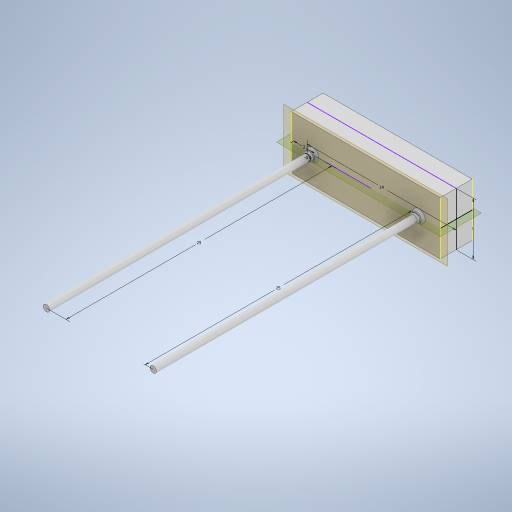
# Autodesk Inventor part: A54
Saved by Autodesk Inventor 2024 (Build 280153000, 153)
## iProperties
Created: 2023-12-15
Part Number: A54
Material: Generic
Document SubType Name: Sheet Metal
Designer: user
Density: 1 g/cm^3
Sheet Metal Rule: Default
Appearance: Default
Author: user
Autodesk Inventor part; units mm, degrees
ref_plane "YZ Plane" through (0, 0, 0) normal (1, 0, 0) x (0, 1, 0)
ref_plane "XZ Plane" through (0, 0, 0) normal (0, 1, 0) x (-1, 0, 0)
ref_plane "XY Plane" through (0, 0, 0) normal (0, 0, 1) x (1, 0, 0)
sketch "Sketch1" plane through (0, 0, 0) normal (0, 0, 1) x (1, 0, 0)
  line L0 (0, 0) -> (14, 0)
  line L1 (14, 0) -> (14, 5)
  line L2 (14, 5) -> (0, 5)
  line L3 (0, 5) -> (0, 0)
  dimension "d39" = 14
  dimension "d40" = 5
  constraints: 8 end point, 1 horizontal, 1 perpendicular
  measures "d39" distance of L0.start L0.end
  measures "d40" distance of L0.end L1.end
extrude "Extrusion1" add sketch "Sketch1" along normal mid plane 3
ref_plane "Work Plane5" through (0, 0, 1.5) normal (0, 0, 1) x (1, 0, 0)
sketch "Sketch9" plane through (0, 0, 1.5) normal (0, 0, 1) x (1, 0, 0)
  line L0 (0, 5) -> (0, 0) projected
  line L1 (0, 2.5) -> (2, 2.5)
  line L2 (14, 0) -> (14, 5) projected
  line L3 (14, 2.5) -> (12, 2.5)
  circle A0 centre (12, 2.5) radius 0.4
  circle A1 centre (2, 2.5) radius 0.4
  dimension "d43" = 2
  dimension "d44" = 2
  dimension "d45" = 0.8
  dimension "d46" = 0.8
  constraints: 4 end point, 2 centre point, 2 coincident, 2 horizontal, 2 midpoint
  measures "d43" distance of L1.start L1.end
  measures "d44" distance of L3.start L3.end
  measures "d45" diameter of A0
  measures "d46" diameter of A1
extrude "Extrusion5" add sketch "Sketch9" along normal blind 0.5
fillet "Fillet5" radius 0.2 4 edges at (11.6, 2.5, 1.5) (11.6, 2.5, 2) (1.6, 2.5, 1.5) (1.6, 2.5, 2)
sketch "Sketch10" plane through (14, 0, 1.5) normal (1, 0, 0) x (0, 0, -1)
  line L0 (3, 5) -> (3, 0) projected
  line L1 (3, 2.5) -> (0, 2.5)
  line L2 (0, 0) -> (0, 5) projected
  point P0 (1.5, 0)
  constraints: 2 end point, 2 midpoint
sketch "Sketch11" plane through (0, 0, 1.5) normal (0, 0, 1) x (1, 0, 0)
  line L0 (14, 0) -> (14, 5) projected
  circle A0 centre (12, 2.5) radius 0.2 projected
  line L1 (7.4995, 2.5) -> (3.1588, 2.5)
  point P0 (0, 0)
  constraints: 2 end point
sketch "Sketch12" plane through (0, 0, 1.5) normal (-1, 0, 0) x (0, 0, 1)
  line L0 (-3, 5) -> (-3, 0) projected
  line L1 (-3, 2.5) -> (0, 2.5)
  line L2 (0, 1.9) -> (0, 3.1) projected
  point P0 (-1.5, 0)
  constraints: 2 end point, 2 midpoint
sketch "Sketch13" plane through (0, 0, 1.5) normal (0, 0, 1) x (1, 0, 0)
  line L0 (0, 5) -> (0, 0) projected
  point P0 (0, 2.5)
  constraints: 1 midpoint
ref_plane "Work Plane7" through (2, 2.5, 2) normal (0, 0, 1) x (1, 0, 0)
ref_plane "Work Plane8" through (12, 2.5, 2) normal (0, 0, 1) x (1, 0, 0)
sketch "Sketch15" plane through (2, 2.5, 2) normal (0, 0, 1) x (1, 0, 0)
  circle A0 centre (0, 0) radius 0.2 projected
  circle A1 centre (0, 0) radius 0.3
  point P0 (-2, -2.5)
  dimension "d57" = 0.6
  constraints: 1 centre point, 1 coincident
  measures "d57" diameter of A1
sketch "Sketch17" plane through (12, 2.5, 2) normal (0, 0, 1) x (1, 0, 0)
  circle A0 centre (0, 0) radius 0.3
  point P0 (-12, -2.5)
  dimension "d63" = 0.6
  constraints: 1 centre point
  measures "d63" diameter of A0
ref_plane "Work Plane9" through (0, 2.5, -1.5) normal (0, -1, 0) x (0, 0, 1)
sketch "Sketch18" plane through (0, 2.5, -1.5) normal (0, -1, 0) x (0, 0, 1)
  line L0 (3, -2) -> (28, -2)
  line L1 (2.9646, -12) -> (27.9646, -12)
  point P0 (1.5, 0)
  point P1 (3, 0)
  dimension "d66" = 2
  dimension "d67" = 25
  dimension "d69" = 25
  constraints: 4 end point
  measures "d66" distance of point (3, 0) L0.start
  measures "d67" distance of L0.start L0.end
  measures "d69" distance of L1.start L1.end
sweep "Sweep6" add profiles "Sketch15" path "Sketch18" path curves L0 contours A0 | A1
sweep "Sweep7" add profiles "Sketch17" path "Sketch18" path curves L1
equation "\"BendRadius\" = Thickness"
equation "\"BendReliefWidth\" = Thickness"
equation "\"BendReliefDepth\" = 0.5 * Thickness"
equation "\"CornerReliefSize\" = 4 * Thickness"
equation "\"MinimumRemnant\" = 2 * Thickness"
equation "\"TransitionRadius\" = BendRadius"
equation "\"JacobiRadiusSize\" = BendRadius"
equation "\"GapSize\" = Thickness"
equation "\"Thickness\" = 3.048"
body "Solid1"
